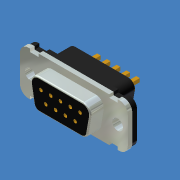
# Autodesk Inventor part: DBConnector
Saved by Autodesk Inventor 2019 (Build 230136000, 136)
## iProperties
Shininess: 64.0
Angle Display Precision: 2
Document Length Units: 11272
Document Angle Units: 11279
Document Time Units: 11290
Document Mass Units: 11286
Document Length Units Precision: 3
Document Angle Units Precision: 2
Compacted: True
Created: 2001-12-01
Part Number: DBConnector
Description: Dsub 9 Pin, 2 Row, Female
Document SubType Name: Modeling
Designer: Charles Bliss
Material: Generic
Density: 1 g/cm^3
Appearance: Zinc
Density: 0.0
Volumn: 0.0
Area: 0.0
PropertySet Name: Model Information
Control State: 0
Master: False
Checked Out: False
Author: Charles Bliss
Autodesk Inventor part; units mm, degrees
ref_plane "YZ Plane" through (0, 0, 0) normal (1, 0, 0) x (0, 1, 0)
ref_plane "XZ Plane" through (0, 0, 0) normal (0, 1, 0) x (-1, 0, 0)
ref_plane "XY Plane" through (0, 0, 0) normal (0, 0, 1) x (1, 0, 0)
sketch "Sketch1" plane through (0, 0, 0) normal (0, 0, 1) x (1, 0, 0)
  line L0 (-10.0784, 6.2738) -> (10.0784, 6.2738)
  line L1 (10.0784, 6.2738) -> (10.0784, 5.4179)
  line L2 (10.0784, 5.4179) -> (12.4968, 5.4179)
  line L3 (12.4968, 5.4179) -> (12.4968, 6.2738)
  line L4 (12.4968, 6.2738) -> (12.9867, 6.2738)
  arc A0 (15.4051, 3.8554) -> (12.9867, 6.2738) centre (12.9867, 3.8554) ccw
  line L5 (-10.0784, 6.2738) -> (-10.0784, 5.4179)
  line L6 (-10.0784, 5.4179) -> (-12.4968, 5.4179)
  line L7 (-12.4968, 5.4179) -> (-12.4968, 6.2738)
  line L8 (-12.4968, 6.2738) -> (-12.9867, 6.2738)
  arc A1 (-12.9867, 6.2738) -> (-15.4051, 3.8554) centre (-12.9867, 3.8554) ccw
  line L9 (-15.4051, 0) -> (15.4051, 0) construction
  line L10 (-10.0784, -6.2738) -> (10.0784, -6.2738)
  line L11 (-10.0784, -6.2738) -> (-10.0784, -5.4179)
  line L12 (-10.0784, -5.4179) -> (-12.4968, -5.4179)
  line L13 (-12.4968, -5.4179) -> (-12.4968, -6.2738)
  line L14 (-12.4968, -6.2738) -> (-12.9867, -6.2738)
  arc A2 (-15.4051, -3.8554) -> (-12.9867, -6.2738) centre (-12.9867, -3.8554) ccw
  line L15 (10.0784, -6.2738) -> (10.0784, -5.4179)
  line L16 (10.0784, -5.4179) -> (12.4968, -5.4179)
  line L17 (12.4968, -5.4179) -> (12.4968, -6.2738)
  line L18 (12.4968, -6.2738) -> (12.9867, -6.2738)
  arc A3 (12.9867, -6.2738) -> (15.4051, -3.8554) centre (12.9867, -3.8554) ccw
  line L19 (-15.4051, 3.8554) -> (-15.4051, -3.8554)
  line L20 (15.4051, 3.8554) -> (15.4051, -3.8554)
  line L21 (-7.7061, -2.9297) -> (-8.5123, 1.6425)
  arc A4 (-6.2567, 4.3307) -> (-8.5123, 1.6425) centre (-6.2567, 2.0403) ccw
  line L22 (-6.2567, 4.3307) -> (6.2567, 4.3307)
  arc A5 (8.5123, 1.6425) -> (6.2567, 4.3307) centre (6.2567, 2.0403) ccw
  line L23 (8.5123, 1.6425) -> (7.7061, -2.9297)
  arc A6 (6.0364, -4.3307) -> (7.7061, -2.9297) centre (6.0364, -2.6353) ccw
  line L24 (6.0364, -4.3307) -> (-6.0364, -4.3307)
  arc A7 (-7.7061, -2.9297) -> (-6.0364, -4.3307) centre (-6.0364, -2.6353) ccw
  line L25 (0, 6.2738) -> (0, -6.2738) construction
  line L26 (0, 4.3307) -> (0, -4.3307) construction
  line L27 (-6.0364, -3.9497) -> (6.0364, -3.9497)
  arc A8 (6.0364, -3.9497) -> (7.3309, -2.8635) centre (6.0364, -2.6353) ccw
  line L28 (7.3309, -2.8635) -> (8.1371, 1.7087)
  arc A9 (8.1371, 1.7087) -> (6.2567, 3.9497) centre (6.2567, 2.0403) ccw
  line L29 (6.2567, 3.9497) -> (-6.2567, 3.9497)
  arc A10 (-6.2567, 3.9497) -> (-8.1371, 1.7087) centre (-6.2567, 2.0403) ccw
  line L30 (-8.1371, 1.7087) -> (-7.3309, -2.8635)
  arc A11 (-7.3309, -2.8635) -> (-6.0364, -3.9497) centre (-6.0364, -2.6353) ccw
  circle A12 centre (-12.4968, 0) radius 1.524
  circle A13 centre (12.4968, 0) radius 1.524
  line L31 (-12.4968, 0) -> (0, 0) construction
  line L32 (0, 0) -> (12.4968, 0) construction
  line L33 (8.1661, 6.2738) -> (8.1661, 2.0403) construction
  line L34 (-8.1661, 6.2738) -> (-8.1661, 2.0403) construction
  line L35 (-8.4735, 1.4224) -> (8.4735, 1.4224) construction
  line L36 (-7.9719, -1.4224) -> (7.9719, -1.4224) construction
  circle A14 centre (-5.588, 1.4224) radius 0.4953
  circle A15 centre (-4.191, -1.4224) radius 0.4953
  line L37 (-7.4703, -4.2672) -> (7.4703, -4.2672) construction
  circle A16 centre (-5.588, -4.2672) radius 0.4953
  point P0 (0, -1.4224)
  dimension "d0" = 10
  dimension "HoleCtr" = 24.9936
  dimension "OAL" = 30.8102
  dimension "ShellLen" = 16.3322
  dimension "ShellWid" = 7.8994
  dimension "HoleDia" = 3.048
  dimension "d6" = 0.381
  dimension "d7" = 2.4184
  dimension "d8" = 0.8559
  dimension "d9" = 2.4184
  dimension "OAW" = 12.5476
  dimension "d11" = 1.3144
  dimension "PinVertDist" = 2.8448
  dimension "PinDia" = 0.9906
  dimension "Pin1Offset" = 5.588
  dimension "d19" = 1.397
  dimension "d34" = 1.9094
  dimension "CLoffset" = 2.5273
  dimension "d52" = 2.8448
  constraints: 76 end point, 26 point on circle, 17 centre point, 16 tangent, 14 point on line, 14 symmetric about line, 10 parallel, 8 midpoint, 6 equal length, 6 equal radius, 5 collinear, 4 perpendicular, 3 horizontal, 3 vertical alignment, 2 coincident, 2 vertical, 18 other
  measures "d0" angle of L21 L19
  measures "HoleCtr" diameter of A12.centre L25
  measures "OAL" distance between parallel lines of L20 L19
  measures "ShellLen" distance between parallel lines of L33 L34
  measures "ShellWid" distance between parallel lines of L27 L29
  measures "HoleDia" diameter of A13
  measures "d6" distance between parallel lines of L30 L21
  measures "d7" distance of L6.start L6.end
  measures "d8" distance of L0.start L6.start
  measures "d9" radius of A1
  measures "OAW" distance between parallel lines of L10 L0
  measures "d11" radius of A8
  measures "PinVertDist" distance between parallel lines of L36 L35
  measures "PinDia" diameter of A15
  measures "Pin1Offset" distance from line of A14.centre L26
  measures "d19" horizontal distance of A15.centre A14.centre
  measures "d34" radius of A10
  measures "CLoffset" distance between parallel lines of L27 L36
  measures "d52" distance between parallel lines of L37 L36
extrude "Extrusion1" add sketch "Sketch1" along normal blind 1.27 contours L0 L1 L2 L3 L4 A0 L20 A3 L18 L17 L16 L15 L10 L11 L12 L13 L14 A2 L19 A1 L8 L7 L6 L5 | L21 A4 L22 A5 L23 A6 L24 A16 L27 A8 L28 A9 L29 A10 L30 A11 A7 | A16 L27 L24 A7 | A7 L24 A16
extrude "Extrusion2" add sketch "Sketch1" along normal blind 5.08 contours L21 A4 L22 A5 L23 A6 L24 A16 L27 A8 L28 A9 L29 A10 L30 A11 A7 | A16 L27 L24 A7
fillet "Fillet4" radius 0.381 8 edges at (-7.1262, -3.934, 5.08) (-8.1092, -0.6436, 5.08) (-8.0112, 3.5125, 5.08) (0, 4.3307, 5.08) (8.0112, 3.5125, 5.08) (8.1092, -0.6436, 5.08) (7.1262, -3.934, 5.08) (0, -4.3307, 5.08)
extrude "Pin1" add sketch "Sketch1" along normal blind 5.08 contours A14
extrude "Pin2" add sketch "Sketch1" along normal blind 5.08 contours A15
extrude "Pin50" [suppressed]
fillet "Fillet1" radius 0.4953 1 edges at (-6.0833, 1.4224, 5.08)
fillet "Fillet2" radius 0.4953 1 edges at (-4.6863, -1.4224, 5.08)
fillet "Fillet50" [suppressed]
sketch "Sketch2" plane through (0, 0, 0) normal (0, 0, -1) x (-1, 0, 0)
  circle A0 centre (-12.4968, 0) radius 1.524 projected
  circle A1 centre (12.4968, 0) radius 1.524 projected
  line L0 (10.0784, 6.2738) -> (-10.0784, 6.2738) projected
  line L1 (-10.0784, 6.2738) -> (-10.0784, 5.4179) projected
  line L2 (-10.0784, 5.4179) -> (-12.4968, 5.4179) projected
  line L3 (-12.4968, 5.4179) -> (-12.4968, 6.2738) projected
  line L4 (-12.4968, 6.2738) -> (-12.9867, 6.2738) projected
  arc A2 (-12.9867, 6.2738) -> (-15.4051, 3.8554) centre (-12.9867, 3.8554) ccw projected
  line L5 (-15.4051, 3.8554) -> (-15.4051, -3.8554) projected
  arc A3 (-15.4051, -3.8554) -> (-12.9867, -6.2738) centre (-12.9867, -3.8554) ccw projected
  line L6 (-12.9867, -6.2738) -> (-12.4968, -6.2738) projected
  line L7 (-12.4968, -6.2738) -> (-12.4968, -5.4179) projected
  line L8 (-12.4968, -5.4179) -> (-10.0784, -5.4179) projected
  line L9 (-10.0784, -5.4179) -> (-10.0784, -6.2738) projected
  line L10 (-10.0784, -6.2738) -> (10.0784, -6.2738) projected
  line L11 (10.0784, -6.2738) -> (10.0784, -5.4179) projected
  line L12 (10.0784, -5.4179) -> (12.4968, -5.4179) projected
  line L13 (12.4968, -5.4179) -> (12.4968, -6.2738) projected
  line L14 (12.4968, -6.2738) -> (12.9867, -6.2738) projected
  arc A4 (12.9867, -6.2738) -> (15.4051, -3.8554) centre (12.9867, -3.8554) ccw projected
  line L15 (15.4051, -3.8554) -> (15.4051, 3.8554) projected
  arc A5 (15.4051, 3.8554) -> (12.9867, 6.2738) centre (12.9867, 3.8554) ccw projected
  line L16 (12.9867, 6.2738) -> (12.4968, 6.2738) projected
  line L17 (12.4968, 6.2738) -> (12.4968, 5.4179) projected
  line L18 (12.4968, 5.4179) -> (10.0784, 5.4179) projected
  line L19 (10.0784, 5.4179) -> (10.0784, 6.2738) projected
  line L20 (-9.8244, 6.0198) -> (9.8244, 6.0198)
  line L21 (9.8244, 6.0198) -> (9.8244, 5.1639)
  line L22 (9.8244, 5.1639) -> (12.7508, 5.1639)
  line L23 (12.7508, 5.1639) -> (12.7508, 6.0198)
  line L24 (12.7508, 6.0198) -> (12.9867, 6.0198)
  arc A6 (15.1511, 3.8554) -> (12.9867, 6.0198) centre (12.9867, 3.8554) ccw
  line L25 (15.1511, 3.8554) -> (15.1511, -3.8554)
  arc A7 (12.9867, -6.0198) -> (15.1511, -3.8554) centre (12.9867, -3.8554) ccw
  line L26 (12.9867, -6.0198) -> (12.7508, -6.0198)
  line L27 (12.7508, -6.0198) -> (12.7508, -5.1639)
  line L28 (12.7508, -5.1639) -> (9.8244, -5.1639)
  line L29 (9.8244, -5.1639) -> (9.8244, -6.0198)
  line L30 (9.8244, -6.0198) -> (-9.8244, -6.0198)
  line L31 (-9.8244, -6.0198) -> (-9.8244, -5.1639)
  line L32 (-9.8244, -5.1639) -> (-12.7508, -5.1639)
  line L33 (-12.7508, -5.1639) -> (-12.7508, -6.0198)
  line L34 (-12.7508, -6.0198) -> (-12.9867, -6.0198)
  arc A8 (-15.1511, -3.8554) -> (-12.9867, -6.0198) centre (-12.9867, -3.8554) ccw
  line L35 (-15.1511, -3.8554) -> (-15.1511, 3.8554)
  arc A9 (-12.9867, 6.0198) -> (-15.1511, 3.8554) centre (-12.9867, 3.8554) ccw
  line L36 (-12.9867, 6.0198) -> (-12.7508, 6.0198)
  line L37 (-12.7508, 6.0198) -> (-12.7508, 5.1639)
  line L38 (-12.7508, 5.1639) -> (-9.8244, 5.1639)
  line L39 (-9.8244, 5.1639) -> (-9.8244, 6.0198)
  dimension "d35" = 0.254
  constraints: 40 end point, 8 point on circle, 4 centre point, 23 other
  measures "d35" distance between parallel lines of L5 L35
extrude "Extrusion5" add sketch "Sketch2" along normal blind 1.6002 contours L20 L21 L22 L23 L24 A6 L25 A7 L26 L27 L28 L29 L30 L31 L32 L33 L34 A8 L35 A9 L36 L37 L38 L39
sketch "Sketch3" plane through (0, 0, -1.6002) normal (0, 0, -1) x (-1, 0, 0)
  line L0 (-7.5557, 5.2197) -> (7.5557, 5.2197)
  arc A0 (9.4361, 2.9787) -> (7.5557, 5.2197) centre (7.5557, 3.3103) ccw
  line L1 (9.4361, 2.9787) -> (8.2687, -3.6418)
  arc A1 (6.3883, -5.2197) -> (8.2687, -3.6418) centre (6.3883, -3.3103) ccw
  line L2 (6.3883, -5.2197) -> (-6.3883, -5.2197)
  arc A2 (-8.2687, -3.6418) -> (-6.3883, -5.2197) centre (-6.3883, -3.3103) ccw
  line L3 (-8.2687, -3.6418) -> (-9.4361, 2.9787)
  arc A3 (-7.5557, 5.2197) -> (-9.4361, 2.9787) centre (-7.5557, 3.3103) ccw
  line L4 (0, 0) -> (0, 5.2197) construction
  line L5 (0, 0) -> (0, -5.2197) construction
  line L6 (-9.8244, 6.0198) -> (9.8244, 6.0198) projected
  line L7 (-8.5123, 1.6425) -> (-7.7061, -2.9297) projected
  dimension "d86" = 1.9094
  dimension "d87" = 10.4394
  dimension "d88" = 18.8722
  constraints: 12 end point, 8 point on circle, 8 tangent, 4 centre point, 2 equal length, 2 horizontal alignment, 2 midpoint, 2 vertical, 1 equal radius, 1 parallel, 1 perpendicular
  measures "d86" radius of A2
  measures "d87" distance of L5.end L4.end
  measures "d88" distance of L1.start L3.end
extrude "Extrusion6" add sketch "Sketch3" along normal blind 5.08
sketch "Sketch4" plane through (0, 0, -6.6802) normal (0, 0, -1) x (-1, 0, 0)
  line L0 (3.683, -0.9144) -> (4.699, -0.9144)
  line L1 (4.699, -0.9144) -> (4.699, -1.9304)
  line L2 (4.699, -1.9304) -> (3.683, -1.9304)
  line L3 (3.683, -1.9304) -> (3.683, -0.9144)
  line L4 (5.08, 1.9304) -> (6.096, 1.9304)
  line L5 (6.096, 1.9304) -> (6.096, 0.9144)
  line L6 (6.096, 0.9144) -> (5.08, 0.9144)
  line L7 (5.08, 0.9144) -> (5.08, 1.9304)
  line L8 (6.096, -4.7752) -> (5.08, -4.7752)
  line L9 (5.08, -4.7752) -> (5.08, -3.7592)
  line L10 (5.08, -3.7592) -> (6.096, -3.7592)
  line L11 (6.096, -3.7592) -> (6.096, -4.7752)
  point P0 (5.588, 1.4224)
  point P1 (4.191, -1.4224)
  point P2 (4.191, -1.4224)
  point P3 (5.588, 1.4224)
  point P4 (5.588, -4.2672)
  point P5 (5.588, -4.2672)
  dimension "d46" = 1.016
  constraints: 24 end point, 3 coincident, 3 horizontal, 2 parallel, 21 other
  measures "d46" distance of L4.end L5.end
extrude "Extrusion7" add sketch "Sketch4" along normal blind 5.08 contours L0 L1 L2 L3
extrude "Extrusion8" add sketch "Sketch4" along normal blind 5.08 contours L4 L5 L6 L7
extrude "ExtrudeSgr50" [suppressed]
chamfer "Chamfer1" distance 0.3048 angle 45 4 edges at (-5.588, 0.9144, -11.7602) (-5.08, 1.4224, -11.7602) (-5.588, 1.9304, -11.7602) (-6.096, 1.4224, -11.7602)
chamfer "Chamfer2" distance 0.3048 angle 45 4 edges at (-3.683, -1.4224, -11.7602) (-4.191, -0.9144, -11.7602) (-4.699, -1.4224, -11.7602) (-4.191, -1.9304, -11.7602)
chamfer "Chamfer50" [suppressed]
pattern_linear "Pattern1" count 5 spacing 2.794 along (1, 0, 0) of "Pin1", "Extrusion8", "Fillet1", "Chamfer1"
pattern_linear "Pattern2" count 4 spacing 2.794 along (1, 0, 0) of "Pin2", "Extrusion7", "Fillet2", "Chamfer2"
pattern_linear "Pattern50" [suppressed]
pattern_linear "Pattern15" [suppressed]
extrude "Female" add sketch "Sketch1" along normal blind 5.1054 contours A16 L27 | L27 A11 L30 A10 L29 A9 L28 A8 A16 | A14 | A15
extrude "Socket1" cut sketch "Sketch1" along normal through all contours A14
extrude "Socket2" cut sketch "Sketch1" along normal through all contours A15
extrude "Socket50" [suppressed]
pattern_linear "Pattern5" count 5 spacing 2.794 along (1, 0, 0) of "Socket1"
pattern_linear "Pattern6" count 4 spacing 2.794 along (1, 0, 0) of "Socket2"
pattern_linear "Pattern7" [suppressed]
equation "\"d19\" = 0.5 * PinSpace"
equation "\"d52\" = PinVertDist"
equation "\"d63\" = d6"
equation "\"d26\" = d24"
equation "\"d53\" = d24"
equation "\"d44\" = 0.5 * PinDia"
equation "\"d45\" = 0.5 * PinDia"
equation "\"d55\" = 0.5 * PinDia"
equation "\"d56\" = d24"
equation "\"d47\" = 0.3 * d46"
equation "\"d48\" = 0.3 * d46"
equation "\"d49\" = 0.3 * d46"
equation "\"d50\" = 0.3 * d46"
equation "\"d58\" = 0.2 * d46"
equation "\"d59\" = 0.2 * d46"
equation "\"d30\" = PinSpace"
equation "\"d33\" = PinSpace"
equation "\"d62\" = PinSpace"
equation "\"d66\" = PinSpace"
equation "\"d77\" = PinSpace"
equation "\"d80\" = PinSpace"
equation "\"d83\" = PinSpace"
equation "\"PinSpace\" = 2.794"
equation "\"RowOffset\" = 1.397"
equation "\"d24\" = 5.08"
body "Solid1"
